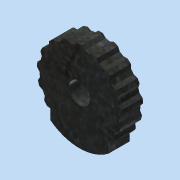
# Autodesk Inventor part: Wheel
Saved by Autodesk Inventor 2015 (Build 190159000, 159)
## iProperties
Created: 2015-11-12
Part Number: Wheel
Material: ABS Plastic
Document SubType Name: Modeling
Designer: Raphael
Density: 1.06 g/cm^3
Appearance: Plate
Author: Raphael
Autodesk Inventor part; units mm, degrees
ref_plane "YZ Plane" through (0, 0, 0) normal (1, 0, 0) x (0, 1, 0)
ref_plane "XZ Plane" through (0, 0, 0) normal (0, 1, 0) x (-1, 0, 0)
ref_plane "XY Plane" through (0, 0, 0) normal (0, 0, 1) x (1, 0, 0)
derived "CaseRight.ipt"
sketch "Sketch2" plane through (0, 0, 0) normal (0, 0, 1) x (1, 0, 0)
  circle A0 centre (0, 0) radius 12.7
  circle A1 centre (0, 0) radius 11.9062
  line L0 (-17.78, 0) -> (17.78, 0) projected
  line L1 (0, -17.78) -> (0, 17.78) projected
  line L2 (-0.6647, 12.6826) -> (-1.5541, 11.8044)
  line L3 (1.5541, 11.8044) -> (0.6647, 12.6826)
  circle A2 centre (0, 0) radius 3.175
  dimension "d1" = 25.4
  dimension "d2" = 0.7937
  dimension "d3" = 15
  dimension "d4" = 6
  dimension "d12" = 6.35
  constraints: 4 end point, 4 point on circle, 3 centre point, 3 coincident, 1 other
  measures "d1" diameter of A0
  measures "d2" radial gap between concentric circles of A0 A1
  measures "d12" diameter of A2
extrude "Extrusion1" add sketch "Sketch2" along normal mid plane 6.35 contours L0 A2 L1 A1 | A1 L1 A2 L0 | A1 L0 A2 L1 | L1 A2 L0 A1
extrude "Extrusion2" add sketch "Sketch2" along normal mid plane 6.35 contours L3 A1 L1 A0 | L1 A1 L2 A0
pattern_circular "Circular Pattern1" count 17 over 360 about axis through (0, 0, -10) along (0, 0, 1) of "Extrusion2"
sketch "Sketch3" plane through (0, 0, 3.175) normal (0, 0, 1) x (1, 0, 0)
  line L0 (0, 0) -> (-1.9328, -2.5189) construction
  line L1 (0, 0) -> (1.9328, -2.5189) construction
  arc A0 (-8.6977, -11.335) -> (8.6977, -11.335) centre (0, 0) ccw
  line L2 (0, -20.0025) -> (0, 20.0025) construction
  circle A1 centre (0, 0) radius 3.175 projected
  circle A2 centre (0, 0) radius 3.175
  line L3 (-1.9328, -2.5189) -> (-8.6977, -11.335) construction
  line L4 (1.9328, -2.5189) -> (8.6977, -11.335) construction
  line L5 (-8.6977, -11.335) -> (8.6977, -11.335)
  line L6 (8.6977, -11.335) -> (8.6977, 0)
  line L7 (-8.6977, 0) -> (-8.6977, -11.335)
  line L8 (-20.0025, 0) -> (20.0025, 0) projected
  line L9 (8.6977, 0) -> (3.175, 0)
  line L10 (-3.175, 0) -> (-8.6977, 0)
  dimension "d13" = 75
  dimension "d14" = 28.575
  constraints: 18 end point, 6 point on circle, 4 collinear, 3 parallel, 2 centre point, 2 coincident, 1 concentric, 1 horizontal, 1 perpendicular, 1 other
  measures "d13" angle of L0 L1
  measures "d14" diameter of A0
extrude "Extrusion3" add sketch "Sketch3" against normal up to surface (6.35 mm away) contours L5 A0 | L7 L8 A1 L6 L5
equation "\"d1\" = wheel_diameter"
equation "\"wheel_diameter\" = 25.4"
body "Solid1"
